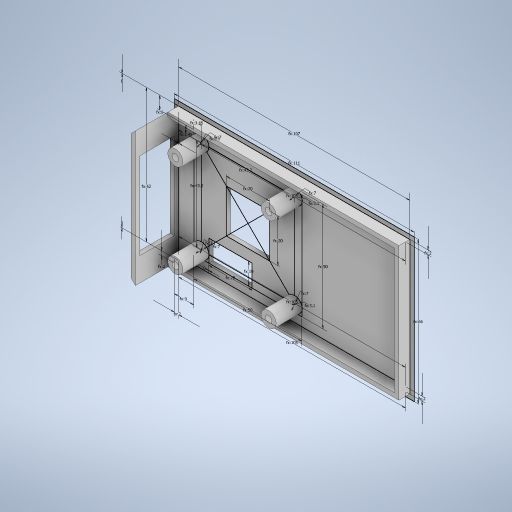
# Autodesk Inventor part: Cap
Saved by Autodesk Inventor 2024 (Build 280153000, 153)
## iProperties
Created: 2024-07-20
Part Number: Cap
Material: Generic
Document SubType Name: Modeling
Designer: Andrei
Density: 1 g/cm^3
Appearance: Default
Author: Andrei
Autodesk Inventor part; units mm, degrees
ref_plane "YZ Plane" through (0, 0, 0) normal (1, 0, 0) x (0, 1, 0)
ref_plane "XZ Plane" through (0, 0, 0) normal (0, 1, 0) x (-1, 0, 0)
ref_plane "XY Plane" through (0, 0, 0) normal (0, 0, 1) x (1, 0, 0)
sketch "Sketch1" plane through (0, 0, 0) normal (0, 0, 1) x (1, 0, 0)
  line L0 (0, 0) -> (111, 0)
  line L1 (111, 0) -> (111, 66)
  line L2 (111, 66) -> (0, 66)
  line L3 (0, 66) -> (0, 0)
  line L4 (2, 2) -> (109, 2)
  line L5 (109, 2) -> (109, 64)
  line L6 (109, 64) -> (2, 64)
  line L7 (2, 64) -> (2, 2)
  line L8 (2, 64) -> (107, 64)
  line L9 (107, 64) -> (107, 2)
  line L10 (107, 2) -> (2, 2)
  line L11 (2, 2) -> (2, 64)
  line L12 (2, 64) -> (0, 64)
  line L13 (0, 64) -> (0, 2)
  line L14 (0, 2) -> (2, 2)
  line L15 (2, 2) -> (2, 64)
  line L16 (2, 64) -> (107, 64)
  line L17 (107, 64) -> (107, 62)
  line L18 (107, 62) -> (2, 62)
  line L19 (2, 62) -> (2, 64)
  line L20 (2, 2) -> (107, 2)
  line L21 (107, 2) -> (107, 4)
  line L22 (107, 4) -> (2, 4)
  line L23 (2, 4) -> (2, 2)
  point P0 (2, 64)
  point P1 (2, 2)
  point P2 (107, 2)
  point P3 (2, 4)
  point P4 (2, 62)
  dimension "d0" = 111
  dimension "d1" = 66
  dimension "d2" = 107
  dimension "d3" = 2
  dimension "d4" = 2
  dimension "d5" = 62
  dimension "d6" = 105
  dimension "d8" = 0
  dimension "d9" = 0
  dimension "d10" = 0
  dimension "d56" = 105
  dimension "d57" = 2
  dimension "d58" = 105
  dimension "d59" = 2
  constraints: 48 end point, 12 parallel, 6 horizontal, 6 perpendicular, 2 point on line
  measures "d0" distance of L2.end L1.end
  measures "d1" distance of L1.end L0.end
  measures "d2" distance of L6.end L5.end
  measures "d3" distance between parallel lines of L7 L3
  measures "d4" distance between parallel lines of L0 L4
  measures "d5" distance of L4.start L6.end
  measures "d6" distance of L9.end L10.end
  measures "d8" distance between parallel lines of L11 L7
  measures "d9" distance between parallel lines of L4 L10
  measures "d10" distance between parallel lines of L8 L6
  measures "d56" distance of L17.end L18.end
  measures "d57" distance between parallel lines of L18 L6
  measures "d58" distance of L22.end L21.end
  measures "d59" distance of L21.end L20.end
extrude "Extrusion1" add sketch "Sketch1" against normal blind 2
extrude "Extrusion2" add sketch "Sketch1" along normal blind 5 contours L9 L6 L5 L4
extrude "Extrusion3" add sketch "Sketch1" along normal blind 20 contours L3 L12 L7 L14
sketch "Sketch2" plane through (0, 0, 0) normal (0, 0, 1) x (1, 0, 0)
  line L0 (9, 58) -> (59, 58)
  line L1 (59, 58) -> (59, 8)
  line L2 (59, 8) -> (9, 8)
  line L3 (9, 8) -> (9, 58)
  line L4 (0, 64) -> (0, 2) projected
  line L5 (2, 64) -> (107, 64) projected
  line L6 (12.45, 54.55) -> (55.65, 54.55)
  line L7 (55.65, 54.55) -> (55.65, 11.35)
  line L8 (55.65, 11.35) -> (12.45, 11.35)
  line L9 (12.45, 11.35) -> (12.45, 54.55)
  circle A0 centre (12.45, 54.55) radius 1.55
  circle A1 centre (55.65, 54.55) radius 1.55
  circle A2 centre (12.45, 11.35) radius 1.55
  circle A3 centre (55.65, 11.35) radius 1.55
  circle A4 centre (12.45, 54.55) radius 3.5
  circle A5 centre (55.65, 54.55) radius 3.5
  circle A6 centre (55.65, 11.35) radius 3.5
  circle A7 centre (12.45, 11.35) radius 3.5
  line L10 (15.95, 18) -> (35.95, 18)
  line L11 (35.95, 18) -> (35.95, 8)
  line L12 (35.95, 8) -> (15.95, 8)
  line L13 (15.95, 8) -> (15.95, 18)
  line L14 (12.45, 54.55) -> (55.65, 11.35)
  line L15 (55.65, 54.55) -> (12.45, 11.35)
  line L16 (24.05, 22.95) -> (44.05, 22.95)
  line L17 (44.05, 22.95) -> (44.05, 42.95)
  line L18 (44.05, 42.95) -> (24.05, 42.95)
  line L19 (24.05, 42.95) -> (24.05, 22.95)
  line L20 (24.05, 22.95) -> (44.05, 42.95) construction
  line L21 (44.05, 22.95) -> (24.05, 42.95) construction
  point P0 (0, 0)
  point P1 (13.0395, 58)
  point P2 (11.8605, 58)
  point P3 (9, 55.1395)
  point P4 (9, 53.9605)
  point P5 (9, 11.9395)
  point P6 (9, 10.7605)
  point P7 (11.4363, 8)
  point P8 (13.4637, 8)
  point P9 (54.6363, 8)
  point P10 (56.6637, 8)
  point P11 (59, 10.3363)
  point P12 (59, 12.3637)
  point P13 (59, 53.5363)
  point P14 (59, 55.5637)
  point P15 (56.2395, 58)
  point P16 (55.0605, 58)
  point P17 (34.05, 32.95)
  dimension "d19" = 50
  dimension "d20" = 50
  dimension "d21" = 9
  dimension "d22" = 6
  dimension "d23" = 43.2
  dimension "d24" = 43.2
  dimension "d25" = 3.45
  dimension "d26" = 3.45
  dimension "d27" = 3.1
  dimension "d28" = 3.1
  dimension "d29" = 3.1
  dimension "d30" = 3.1
  dimension "d31" = 7
  dimension "d32" = 7
  dimension "d33" = 7
  dimension "d34" = 7
  dimension "d47" = 20
  dimension "d48" = 0
  dimension "d49" = 10
  dimension "d50" = 20
  dimension "d51" = 20
  constraints: 40 end point, 8 centre point, 8 coincident, 8 parallel, 4 horizontal, 4 perpendicular, 3 midpoint, 1 point on line
  measures "d19" distance of L1.end L2.end
  measures "d20" distance of L0.end L1.end
  measures "d21" distance between parallel lines of L3 L4
  measures "d22" distance between parallel lines of L0 L5
  measures "d23" distance of L6.end L6.start
  measures "d24" distance of L8.end L6.start
  measures "d25" distance between parallel lines of L6 L0
  measures "d26" distance between parallel lines of L3 L9
  measures "d27" diameter of A0
  measures "d28" diameter of A1
  measures "d29" diameter of A2
  measures "d30" diameter of A3
  measures "d31" diameter of A4
  measures "d32" diameter of A5
  measures "d33" diameter of A6
  measures "d34" diameter of A7
  measures "d47" distance of L11.end L12.end
  measures "d48" distance edge to line of A7 L13
  measures "d49" distance of L10.end L11.end
  measures "d50" distance of L18.end L17.end
  measures "d51" distance of L17.end L16.end
extrude "Extrusion5" add sketch "Sketch2" along normal blind 12 contours A4 L0 | L0 A4 L6 A0 L9 L3 | L3 A4 | A5 L0 | L0 A5 L1 L7 A1 L6 | A4 L14 A0 L6 | A7 L9 A2 L8 L2 L3 | L3 A7 | L9 A0 L14 A4 | L6 A1 L15 A5 | A7 L15 A2 L9 | A5 L1 | L15 A1 L7 A5 | L2 A7 | A7 L8 A2 L15 | A6 L1 | L1 A6 L2 L8 A3 L7 | L7 A3 L14 A6 | L14 A3 L8 A6 | A6 L2
chamfer "Chamfer1" distance 2 angle 45 4 edges at (55.5, 66, -2) (0, 33, -2) (55.5, 0, -2) (111, 33, -2)
sketch "Sketch3" plane through (0, 2, 20) normal (-1, 0, 0) x (0, 0, 1)
  line L0 (-20, 62) -> (0, 62) projected
  line L1 (-20, 62) -> (-20, 0) projected
  line L2 (0, 62) -> (-20, 0)
  line L3 (0, 62) -> (0, 0) projected
  line L4 (0, 0) -> (-20, 62)
  line L5 (-2, 51) -> (-18, 51)
  line L6 (-18, 51) -> (-18, 11)
  line L7 (-18, 11) -> (-2, 11)
  line L8 (-2, 11) -> (-2, 51)
  line L9 (-2, 51) -> (-18, 11) construction
  line L10 (-18, 51) -> (-2, 11) construction
  point P0 (-20, -2)
  point P1 (-15, 62)
  point P2 (-10, 31)
  dimension "d43" = 16
  dimension "d44" = 40
  constraints: 16 end point, 3 midpoint, 2 parallel, 1 horizontal, 1 perpendicular
  measures "d43" distance of L7.end L6.end
  measures "d44" distance of L6.end L5.end
extrude "Extrusion6" cut sketch "Sketch3" along normal mid plane 10 contours L5 L2 L4 | L4 L2 L7 L6 L5 | L5 L8 L7 L4 L2 | L2 L4 L7
extrude "Extrusion7" cut sketch "Sketch2" against normal blind 10 contours L18 L15 L14 | L14 L15 L19 | L17 L14 L15 | L14 L16 L15
extrude "Extrusion8" cut sketch "Sketch2" against normal blind 10 contours L13 L15 L10 L11 L8 | L8 L11 L2 L13 | L13 L10 L15
extrude "Extrusion9" add sketch "Sketch1" along normal blind 5 contours L7 L22 L9 L4 | L6 L9 L18 L7
chamfer "Chamfer3" distance 2 angle 45 2 edges at (0, 2, 10) (0, 64, 10)
equation "\"d0\" = capLength"
equation "\"d1\" = capWidth"
equation "\"d2\" = capLength - 2 * wallWidth"
equation "\"d3\" = wallWidth"
equation "\"d4\" = wallWidth"
equation "\"d5\" = capWidth - 2 * wallWidth"
equation "\"d6\" = capLength - 3 * wallWidth"
equation "\"d56\" = capLength - 3 * wallWidth"
equation "\"d57\" = wallWidth"
equation "\"d58\" = capLength - 3 * wallWidth"
equation "\"d59\" = wallWidth"
equation "\"d11\" = wallWidth"
equation "\"d13\" = wallsHeight"
equation "\"d15\" = height"
equation "\"d19\" = PCBWidth"
equation "\"d20\" = PCBWidth"
equation "\"d21\" = connectorsLength"
equation "\"d22\" = -0.5 * PCBWidth + 0.5 * capWidth - wallWidth"
equation "\"d23\" = widthBetweenHoles"
equation "\"d24\" = widthBetweenHoles"
equation "\"d25\" = holesDistance"
equation "\"d26\" = holesDistance"
equation "\"d27\" = dHoles"
equation "\"d28\" = dHoles"
equation "\"d29\" = dHoles"
equation "\"d30\" = dHoles"
equation "\"d31\" = dBonks"
equation "\"d32\" = dBonks"
equation "\"d33\" = dBonks"
equation "\"d34\" = dBonks"
equation "\"d47\" = cutoutLength"
equation "\"d49\" = cutoutWidth"
equation "\"d50\" = switchersWidth"
equation "\"d51\" = switchersWidth"
equation "\"d43\" = hWindow"
equation "\"d44\" = wWindow"
equation "\"d60\" = wallsHeight"
equation "\"capWidth\" = 66"
equation "\"capLength\" = 111"
equation "\"wallWidth\" = 2"
equation "\"wallsHeight\" = 5"
equation "\"height\" = 20"
equation "\"dHoles\" = 3.1"
equation "\"dBonks\" = 7"
equation "\"PCBWidth\" = 50"
equation "\"connectorsLength\" = 9"
equation "\"widthBetweenHoles\" = 43.2"
equation "\"holesDistance\" = 3.45"
equation "\"hWindowCenter\" = 8"
equation "\"hWindow\" = 16"
equation "\"wWindow\" = 40"
equation "\"cutoutLength\" = 20"
equation "\"cutoutWidth\" = 10"
equation "\"switchersWidth\" = 20"
body "Solid1"
